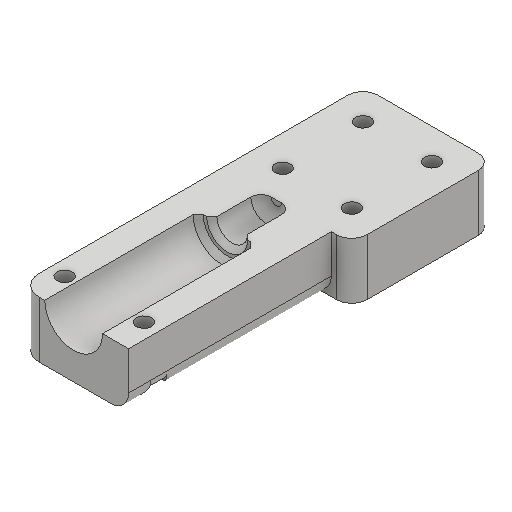
# Autodesk Inventor part: 3DP_ABS_Induction_Sensor_Mount
Saved by Autodesk Inventor 2026.1 (Build 301233000, 233)
## iProperties
Created: 2017-05-27
Part Number: 3DP_ABS_Induction_Sensor_Mount
Material: Ogólny
Document SubType Name: Modeling
Designer: Andrzej
Density: 1 g/cm^3
Appearance: Domyślna
Mass: 14.6301 g
Surface Area: 58.4352 cm^2
Volume: 14.6301 cm^3
Author: Andrzej
Autodesk Inventor part; units mm, degrees
ref_plane "YZ Plane" through (0, 0, 0) normal (1, 0, 0) x (0, 1, 0)
ref_plane "XZ Plane" through (0, 0, 0) normal (0, 1, 0) x (-1, 0, 0)
ref_plane "XY Plane" through (0, 0, 0) normal (0, 0, 1) x (1, 0, 0)
sketch "Szkic1" plane through (0, 0, 0) normal (0, 0, 1) x (1, 0, 0)
  line L0 (-18.7419, 7.0884) -> (6.7581, 7.0884)
  line L1 (6.7581, 7.0884) -> (6.7581, -20.5866)
  line L2 (6.7581, -20.5866) -> (-18.7419, -20.5866)
  line L3 (-18.7419, -20.5866) -> (-18.7419, 7.0884)
  point P0 (0, 0)
  point P1 (-12.7419, 1.0884)
  point P2 (0.7581, 1.0884)
  point P3 (-12.7419, -14.5866)
  point P4 (0.7581, -14.5866)
  dimension "d0" = 15.675
  dimension "d1" = 15.675
  dimension "d2" = 13.5
  dimension "d3" = 13.5
  dimension "d4" = 6
  dimension "d5" = 6
  dimension "d6" = 6
  dimension "d7" = 6
  dimension "d8" = 6
  dimension "d9" = 6
  dimension "d10" = 6
  dimension "d11" = 6
  constraints: 8 end point, 2 parallel, 1 horizontal, 1 perpendicular
  measures "d0" distance of point (-12.742, -14.587) point (-12.742, 1.088)
  measures "d1" distance of point (0.758, -14.587) point (0.758, 1.088)
  measures "d2" distance of point (0.758, 1.088) point (-12.742, 1.088)
  measures "d3" distance of point (0.758, -14.587) point (-12.742, -14.587)
  measures "d4" distance from line of L3 point (-12.742, 1.088)
  measures "d5" distance from line of L3 point (-12.742, -14.587)
  measures "d6" distance from line of L0 point (-12.742, 1.088)
  measures "d7" distance from line of L2 point (-12.742, -14.587)
  measures "d8" distance from line of L0 point (0.758, 1.088)
  measures "d9" distance from line of L2 point (0.758, -14.587)
  measures "d10" distance from line of L1 point (0.758, 1.088)
  measures "d11" distance from line of L1 point (0.758, -14.587)
extrude "Wyciągnięcie proste1" add sketch "Szkic1" along normal blind 27
hole "Otwór1" at (-12.7419, 1.0884, 0) at (0.7581, 1.0884, 0) at (-12.7419, -14.5866, 0) at (0.7581, -14.5866, 0) direction (0, 0, 1) diameter 3 end up to surface
sketch "Szkic2" plane through (-18.7419, -20.5866, 0) normal (0, -1, 0) x (1, 0, 0)
  line L0 (25.5, 0) -> (0, 0) projected
  line L1 (25.5, 0) -> (25.5, 27) projected
  line L2 (0, 27) -> (25.5, 27) projected
  line L3 (0, 0) -> (0, 27) projected
  line L4 (25.5, 27) -> (0, 27) projected
  line L5 (0, 27) -> (21.5, 27)
  line L6 (21.5, 27) -> (21.5, 4.5)
  line L7 (21.5, 4.5) -> (0, 4.5)
  line L8 (0, 4.5) -> (0, 27)
  point P0 (18.7419, 0)
  dimension "d21" = 21.5
  dimension "d22" = 4.5
  constraints: 8 end point, 2 parallel, 1 horizontal, 1 perpendicular
  measures "d21" distance between parallel lines of L6 L3
  measures "d22" distance between parallel lines of L0 L7
extrude "Wyciągnięcie proste2" add sketch "Szkic2" along normal blind 39.625 contours L3 L2 L6 L7
sketch "Szkic4" plane through (0, 0, 27) normal (0, 0, 1) x (1, 0, 0)
  circle A0 centre (-12.7419, -14.5866) radius 1.5 projected
  circle A1 centre (-12.7419, 1.0884) radius 1.5 projected
  circle A2 centre (0.7581, 1.0884) radius 1.5 projected
  circle A3 centre (0.7581, -14.5866) radius 1.5 projected
  line L0 (6.7581, 7.0884) -> (-18.7419, 7.0884) projected
  line L1 (-18.7419, 7.0884) -> (-18.7419, -60.2116) projected
  line L2 (2.7581, -60.2116) -> (-18.7419, -60.2116) projected
  line L3 (2.7581, -20.5866) -> (2.7581, -60.2116) projected
  line L4 (2.7581, -20.5866) -> (6.7581, -20.5866) projected
  line L5 (6.7581, -20.5866) -> (6.7581, 7.0884) projected
  point P0 (0, 0)
extrude "Wyciągnięcie proste4" cut sketch "Szkic4" against normal blind 11.5
fillet "Zaokrąglenie1" radius 3.5 1 edges at (2.7581, -40.3991, 4.5)
sketch "Szkic5" plane through (-18.7419, -60.2116, 0) normal (0, -1, 0) x (1, 0, 0)
  arc A0 (18, 4.5) -> (21.5, 8) centre (18, 8) ccw projected
  line L0 (21.5, 8) -> (21.5, 15.5) projected
  line L1 (21.5, 15.5) -> (0, 15.5) projected
  line L2 (0, 15.5) -> (0, 4.5) projected
  line L3 (0, 4.5) -> (18, 4.5) projected
  line L4 (21.5, 15.5) -> (0, 15.5) projected
  circle A1 centre (10.75, 15.5) radius 5.65
  point P0 (18.7419, 0)
  dimension "d35" = 11.3
  dimension "d36" = 21.5
  constraints: 1 centre point, 1 midpoint
  measures "d35" diameter of A1
  measures "d36" distance between parallel lines of L0 L2
extrude "Wyciągnięcie proste5" cut sketch "Szkic5" against normal blind 30 contours A1 L1 | L1 A1
sketch "Szkic6" plane through (0, 0, 15.5) normal (0, 0, 1) x (1, 0, 0)
  line L0 (-13.6419, -60.2116) -> (-13.6419, -30.2116) projected
  line L1 (-13.6419, -30.2116) -> (-2.3419, -30.2116) projected
  line L2 (-2.3419, -30.2116) -> (-2.3419, -60.2116) projected
  line L3 (2.7581, -60.2116) -> (-2.3419, -60.2116) projected
  line L4 (2.7581, -20.5866) -> (2.7581, -60.2116) projected
  line L5 (6.7581, -20.5866) -> (2.7581, -20.5866) projected
  line L6 (6.7581, 7.0884) -> (6.7581, -20.5866) projected
  line L7 (-18.7419, 7.0884) -> (6.7581, 7.0884) projected
  line L8 (-18.7419, -60.2116) -> (-18.7419, 7.0884) projected
  line L9 (-13.6419, -60.2116) -> (-18.7419, -60.2116) projected
  circle A0 centre (-12.7419, -14.5866) radius 1.5 projected
  circle A1 centre (-12.7419, 1.0884) radius 1.5 projected
  circle A2 centre (0.7581, 1.0884) radius 1.5 projected
  circle A3 centre (0.7581, -14.5866) radius 1.5 projected
  point P0 (0, 0)
  point P1 (-15.7419, -54.2116)
  point P2 (-0.2419, -54.2116)
  dimension "d39" = 5.1
  dimension "d40" = 5.1
  dimension "d41" = 6
  dimension "d42" = 6
  dimension "d43" = 3
  dimension "d44" = 3
  measures "d39" distance between parallel lines of L0 L8
  measures "d40" distance of L3.start L2.end
  measures "d41" distance from line of L9 point (-15.742, -54.212)
  measures "d42" distance from line of L3 point (-0.242, -54.212)
  measures "d43" distance from line of L8 point (-15.742, -54.212)
  measures "d44" distance from line of L4 point (-0.242, -54.212)
hole "Otwór2" at (-15.7419, -54.2116, 15.5) at (-0.2419, -54.2116, 15.5) direction (0, 0, -1) diameter 3 end through all
sketch "Szkic7" plane through (-18.7419, -60.2116, 4.5) normal (0, 0, -1) x (-1, 0, 0)
  arc A0 (-18, 4.5858) -> (-18, 7.4142) centre (-18.5, 6) ccw projected
  line L0 (-18, 0) -> (-18, 4.5858) projected
  line L1 (0, 0) -> (-18, 0) projected
  line L2 (0, 39.625) -> (0, 0) projected
  line L3 (-18, 39.625) -> (0, 39.625) projected
  line L4 (-18, 7.4142) -> (-18, 39.625) projected
  circle A1 centre (-3, 6) radius 1.5 projected
  circle A2 centre (-3, 6) radius 2.85
  circle A3 centre (-18.5, 6) radius 2.85
  line L5 (-0.15, 4.3546) -> (-3, 2.7091)
  line L6 (-3, 2.7091) -> (-5.85, 4.3546)
  line L7 (-5.85, 4.3546) -> (-5.85, 7.6454)
  line L8 (-5.85, 7.6454) -> (-3, 9.2909)
  line L9 (-3, 9.2909) -> (-0.15, 7.6454)
  line L10 (-0.15, 7.6454) -> (-0.15, 4.3546)
  line L11 (-21.35, 7.6454) -> (-18.5, 9.2909)
  line L12 (-18.5, 9.2909) -> (-15.65, 7.6454)
  line L13 (-15.65, 7.6454) -> (-15.65, 4.3546)
  line L14 (-15.65, 4.3546) -> (-18.5, 2.7091)
  line L15 (-18.5, 2.7091) -> (-21.35, 4.3546)
  line L16 (-21.35, 4.3546) -> (-21.35, 7.6454)
  point P0 (-18.7419, 60.2116)
  point P1 (-0.15, 6)
  point P2 (-21.35, 6)
  dimension "d52" = 5.7
  dimension "d53" = 5.7
  constraints: 24 end point, 4 coincident, 2 horizontal alignment, 2 midpoint, 30 other
extrude "Wyciągnięcie proste6" cut sketch "Szkic7" against normal blind 5 contours L0 A3 L4 A0 | A0 L4 A3 L0 | A3 L14 L0 | L0 L14 L15 A3 | A3 L11 L12 L4 | L4 L12 A3 | L15 L16 A3 | A3 L13 L14 | L12 L13 A3 | A3 L16 L11 | A2 | L10 L5 A2 | A2 L9 L10 | A2 L8 L9 | L5 L6 A2 | A2 L7 L8 | L6 L7 A2
sketch "Szkic8" plane through (-18.7419, -30.2116, 0) normal (0, -1, 0) x (1, 0, 0)
  line L0 (5.1, 15.5) -> (16.4, 15.5) projected
  arc A0 (5.1, 15.5) -> (16.4, 15.5) centre (10.75, 15.5) ccw projected
  circle A1 centre (10.75, 15.5) radius 3
  point P0 (18.7419, 0)
  dimension "d56" = 6
  constraints: 1 centre point, 1 coincident
  measures "d56" diameter of A1
extrude "Wyciągnięcie proste7" cut sketch "Szkic8" against normal up to surface (9.625 mm away) contours A1 L0 | L0 A1
chamfer "Faza1" distance 1 angle 45 2 edges at (-7.9919, -30.2116, 9.85) (-7.9919, -30.2116, 12.5)
fillet "Zaokrąglenie2" radius 2 1 edges at (-7.9919, -20.5866, 12.5)
fillet "Zaokrąglenie3" radius 4 1 edges at (-18.7419, -60.2116, 10)
fillet "Zaokrąglenie4" radius 3 3 edges at (6.7581, -20.5866, 7.75) (6.7581, 7.0884, 7.75) (-18.7419, 7.0884, 7.75)
sketch "Szkic9" plane through (0, 0, 0) normal (0, 0, -1) x (-1, 0, 0)
  arc A0 (18.7419, 4.0884) -> (15.7419, 7.0884) centre (15.7419, 4.0884) ccw projected
  line L0 (15.7419, 7.0884) -> (-3.7581, 7.0884) projected
  arc A1 (-3.7581, 7.0884) -> (-6.7581, 4.0884) centre (-3.7581, 4.0884) ccw projected
  line L1 (-6.7581, 4.0884) -> (-6.7581, -17.5866) projected
  arc A2 (-6.7581, -17.5866) -> (-3.7581, -20.5866) centre (-3.7581, -17.5866) ccw projected
  line L2 (-3.7581, -20.5866) -> (18.7419, -20.5866) projected
  line L3 (18.7419, -20.5866) -> (18.7419, 4.0884) projected
  circle A3 centre (12.7419, -14.5866) radius 1.5 projected
  circle A4 centre (12.7419, 1.0884) radius 1.5 projected
  circle A5 centre (-0.7581, 1.0884) radius 1.5 projected
  circle A6 centre (-0.7581, -14.5866) radius 1.5 projected
  point P0 (0, 0)
extrude "Wyciągnięcie proste8" cut sketch "Szkic9" against normal blind 4.5
equation "\"d1\" = d0"
equation "\"d3\" = d2"
equation "\"d8\" = d6"
equation "\"d44\" = d43"
